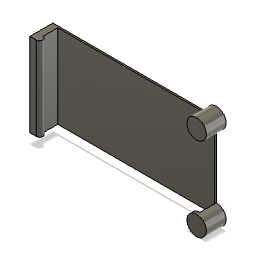
ArduinoMountPlate (Autodesk Fusion 360 design; units mm, degrees)
Autodesk Fusion 360 part; units mm, degrees
sketch "Sketch1" plane through (0, 0, 0) normal (0, 0, 1) x (1, 0, 0)
  line L0 (0, 0) -> (48.35, 0)
  line L1 (48.35, 0) -> (48.35, 25.75)
  line L2 (48.35, 25.75) -> (0, 25.75)
  line L3 (0, 25.75) -> (0, 0)
  line L4 (51.35, 22.75) -> (45.35, 22.75)
  line L5 (45.35, 22.75) -> (45.35, 28.75)
  line L6 (45.35, 28.75) -> (51.35, 28.75)
  line L7 (51.35, 28.75) -> (51.35, 22.75)
  line L8 (51.35, 22.75) -> (45.35, 28.75) construction
  line L9 (45.35, 22.75) -> (51.35, 28.75) construction
  line L10 (51.35, -3) -> (45.35, -3)
  line L11 (45.35, -3) -> (45.35, 3)
  line L12 (45.35, 3) -> (51.35, 3)
  line L13 (51.35, 3) -> (51.35, -3)
  line L14 (51.35, -3) -> (45.35, 3) construction
  line L15 (45.35, -3) -> (51.35, 3) construction
  line L16 (0, 0) -> (-2, 0)
  line L17 (-2, 0) -> (-2, 25.75)
  line L18 (-2, 25.75) -> (0, 25.75)
  line L19 (0, 25.75) -> (0, 0)
  point P0 (48.35, 25.75)
  point P1 (48.35, 0)
  dimension "d1" = 48.35
  dimension "d2" = 25.75
  dimension "d3" = 6
  dimension "d4" = 6
  dimension "d5" = 6
  dimension "d6" = 6
  dimension "d7" = 2
  dimension "d8" = 25.75
  constraint horizontal L0
  constraint vertical L1
  constraint horizontal L2
  constraint vertical L3
  constraint coincident L0.start L3.end
  constraint horizontal L4
  constraint perpendicular L4 L5
  constraint parallel L4 L6
  constraint parallel L5 L7
  constraint coincident L8 P0
  constraint coincident L9 P0
  constraint coincident P0 L1.end
  constraint horizontal L10
  constraint perpendicular L10 L11
  constraint parallel L10 L12
  constraint parallel L11 L13
  constraint coincident L14 P1
  constraint coincident L15 P1
  constraint coincident P1 L0.end
  constraint horizontal L16
  constraint vertical L17
  constraint horizontal L18
  constraint vertical L19
  measures "d1" distance of L0.start L0.end
  measures "d2" distance of L0.start L2.end
  measures "d3" distance of L5.end L6.end
  measures "d4" distance of L4.end L5.end
  measures "d5" distance of L11.end L12.end
  measures "d6" distance of L10.end L11.end
  measures "d7" distance of L0.start L16.end
  measures "d8" distance of L0.start L2.end
extrude "Extrude1" add sketch "Sketch1" along normal blind 0.5
extrude "Extrude2" add sketch "Sketch1" along normal blind 5.1 contours L3 L16 L17 L18 L19
sketch "Sketch2" plane through (0, 0, 5.1) normal (0, 0, 1) x (1, 0, 0)
  line L0 (0, 25.75) -> (-2, 25.75)
  line L1 (-2, 25.75) -> (-2, 0)
  line L2 (-2, 0) -> (0, 0)
  line L3 (0, 0) -> (0, 25.75)
  line L4 (-2, 25.75) -> (1, 25.75)
  line L5 (1, 25.75) -> (1, 0.05)
  line L6 (1, 0.05) -> (-2, 0.05)
  line L7 (-2, 0.05) -> (-2, 25.75)
  dimension "d13" = 3
  dimension "d14" = 25.7
  constraint horizontal L4
  constraint vertical L5
  constraint horizontal L6
  constraint vertical L7
  constraint coincident L0.end L1.start
  measures "d13" distance of L0.end L4.end
  measures "d14" distance of L0.end L6.end
extrude "Extrude3" add sketch "Sketch2" along normal blind 2 contours L0 L1 L3 L4 L6 L7 | L3 L4 L5 L6
fillet "Fillet1" radius 1 2 edges at (1, 12.9, 7.1) (1, 12.9, 5.1)
extrude "Extrude4" add sketch "Sketch1" along normal blind 5.1 contours L0 L1 L10 L11 L12 L13 | L1 L2 L4 L5 L6 L7
sketch "Sketch3" plane through (0, 0, 5.1) normal (0, 0, 1) x (1, 0, 0)
  line L0 (51.35, 3) -> (48.35, 3)
  line L1 (48.35, 3) -> (48.35, 0)
  line L2 (48.35, 0) -> (45.35, 0)
  line L3 (45.35, 0) -> (45.35, -3)
  line L4 (45.35, -3) -> (51.35, -3)
  line L5 (51.35, -3) -> (51.35, 3)
  line L6 (51.35, -3) -> (45.35, -3)
  line L7 (45.35, -3) -> (45.35, 3)
  line L8 (45.35, 3) -> (51.35, 3)
  line L9 (51.35, 3) -> (51.35, -3)
  line L10 (51.35, 28.75) -> (45.35, 28.75)
  line L11 (45.35, 28.75) -> (45.35, 22.75)
  line L12 (45.35, 22.75) -> (51.35, 22.75)
  line L13 (51.35, 22.75) -> (51.35, 28.75)
  point P0 (51.35, 28.75)
  dimension "d21" = 6
  dimension "d22" = 6
  dimension "d23" = 6
  dimension "d24" = 6
  constraint horizontal L6
  constraint vertical L7
  constraint horizontal L8
  constraint vertical L9
  constraint coincident L4.end L5.start
  constraint horizontal L10
  constraint vertical L11
  constraint horizontal L12
  constraint vertical L13
  constraint coincident P0 L10.start
  measures "d21" distance of L4.end L3.end
  measures "d22" distance of L4.end L0.start
  measures "d23" distance of P0 L10.end
  measures "d24" distance of P0 L12.end
extrude "Extrude5" add sketch "Sketch3" along normal blind 1
fillet "Fillet2" radius 3 6 edges at (51.35, -3, 3.05) (51.35, 3, 3.05) (45.35, -3, 3.05) (51.35, 22.75, 3.05) (45.35, 28.75, 3.05) (51.35, 28.75, 3.05)
fillet "Fillet3" radius 3 2 edges at (45.35, 22.75, 5.6) (45.35, 3, 5.6)
